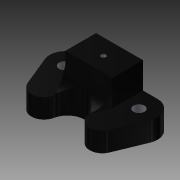
# Autodesk Inventor part: FrontStopper
Saved by Autodesk Inventor 2015 (Build 190159000, 159)
## iProperties
Created: 2017-01-04
Part Number: FrontStopper
Material: Generic
Document SubType Name: Modeling
Designer: Ernest
Density: 1 g/cm^3
Appearance: Default
Author: Ernest
Autodesk Inventor part; units mm, degrees
ref_plane "YZ Plane" through (0, 0, 0) normal (1, 0, 0) x (0, 1, 0)
ref_plane "XZ Plane" through (0, 0, 0) normal (0, 1, 0) x (-1, 0, 0)
ref_plane "XY Plane" through (0, 0, 0) normal (0, 0, 1) x (1, 0, 0)
sketch "Sketch1" plane through (0, 0, 0) normal (0, 0, 1) x (1, 0, 0)
  circle A0 centre (0, 0) radius 8
  circle A1 centre (25.5147, 5) radius 3
  circle A2 centre (-25.5147, 5) radius 3
  circle A3 centre (32.5, 30) radius 5
  circle A4 centre (-32.5, 30) radius 5
  arc A5 (45.4578, 24.6994) -> (32.5, 44) centre (32.5, 30) ccw
  arc A6 (-32.5, 44) -> (-45.4578, 24.6994) centre (-32.5, 30) ccw
  line L0 (-24.3676, 0) -> (22.7562, 0) construction
  line L1 (-38.3266, 30) -> (45.5284, 30) construction
  line L2 (-33.7528, 8) -> (48.0284, 8) construction
  circle A7 centre (-25.5147, 5) radius 6
  circle A8 centre (25.5147, 5) radius 6
  arc A9 (14.72, 2.8846) -> (-15, 0) centre (0, 0) ccw
  arc A10 (-35.6958, 0.8353) -> (-14.72, 2.8846) centre (-25.5147, 5) ccw
  arc A11 (14.72, 2.8846) -> (35.6958, 0.8353) centre (25.5147, 5) ccw
  line L3 (-45.4578, 24.6994) -> (-35.6958, 0.8353)
  line L4 (35.6958, 0.8353) -> (45.4578, 24.6994)
  line L5 (-32.5, 44) -> (32.5, 44)
  dimension "d0" = 65
  dimension "d1" = 32.5
  dimension "d2" = 10
  dimension "d3" = 10
  dimension "d4" = 6
  dimension "d5" = 6
  dimension "d6" = 28
  dimension "d7" = 28
  dimension "d14" = 16
  dimension "d16" = 15
  dimension "d18" = 12
  dimension "d19" = 12
  dimension "d20" = 30
  dimension "d33" = 30
  dimension "d34" = 15
  constraints: 12 centre point, 12 end point, 11 point on circle, 10 tangent, 8 coincident, 4 horizontal, 4 point on line, 2 parallel
  measures "d0" distance of A3.centre A4.centre
  measures "d1" horizontal distance of point (0, 0) A4.centre
  measures "d2" diameter of A4
  measures "d3" diameter of A3
  measures "d4" diameter of A2
  measures "d5" diameter of A1
  measures "d6" diameter of A5
  measures "d7" diameter of A6
  measures "d14" diameter of A0
  measures "d18" diameter of A7
  measures "d19" diameter of A8
  measures "d20" diameter of A9
  measures "d33" distance from line of point (0, 0) L1
extrude "Extrusion1" add sketch "Sketch1" along normal blind 12 contours L4 A11 A9 A10 L3 A6 L5 A5 | A7 | A8
sketch "Sketch2" plane through (0, 0, 12) normal (0, 0, 1) x (1, 0, 0)
  circle A0 centre (25.5147, 5) radius 3 projected
  circle A1 centre (-25.5147, 5) radius 3 projected
  circle A2 centre (-32.5, 30) radius 5 projected
  circle A3 centre (32.5, 30) radius 5 projected
  line L0 (-45.4578, 24.6994) -> (-35.6958, 0.8353) projected
  arc A4 (-35.6958, 0.8353) -> (-14.72, 2.8846) centre (-25.5147, 5) ccw projected
  arc A5 (14.72, 2.8846) -> (-14.72, 2.8846) centre (0, 0) ccw projected
  arc A6 (14.72, 2.8846) -> (35.6958, 0.8353) centre (25.5147, 5) ccw projected
  line L1 (35.6958, 0.8353) -> (45.4578, 24.6994) projected
  arc A7 (45.4578, 24.6994) -> (32.5, 44) centre (32.5, 30) ccw projected
  line L2 (32.5, 44) -> (-32.5, 44) projected
  arc A8 (-32.5, 44) -> (-45.4578, 24.6994) centre (-32.5, 30) ccw projected
  circle A9 centre (-32.5, 30) radius 5 projected
  circle A10 centre (-32.5, 30) radius 7.5
  circle A11 centre (32.5, 30) radius 5
  constraints: 2 centre point, 2 coincident, 1 concentric
extrude "Extrusion2" add sketch "Sketch2" along normal blind 5 contours A0 | A1 | A8 L2 A7 L1 A6 A5 A4 L0 | A10
sketch "Sketch3" plane through (0, 0, 17) normal (0, 0, 1) x (1, 0, 0)
  line L0 (-17.5, 40.5) -> (17.5, 40.5)
  line L1 (17.5, 40.5) -> (17.5, 18.5)
  line L2 (17.5, 18.5) -> (-17.5, 18.5)
  line L3 (-17.5, 18.5) -> (-17.5, 40.5)
  circle A0 centre (32.5, 30) radius 5 projected
  circle A1 centre (-32.5, 30) radius 5 projected
  line L4 (-45.4578, 24.6994) -> (-35.6958, 0.8353) projected
  arc A2 (-35.6958, 0.8353) -> (-14.72, 2.8846) centre (-25.5147, 5) ccw projected
  arc A3 (14.72, 2.8846) -> (-14.72, 2.8846) centre (0, 0) ccw projected
  arc A4 (14.72, 2.8846) -> (35.6958, 0.8353) centre (25.5147, 5) ccw projected
  line L5 (35.6958, 0.8353) -> (45.4578, 24.6994) projected
  arc A5 (45.4578, 24.6994) -> (32.5, 44) centre (32.5, 30) ccw projected
  line L6 (32.5, 44) -> (-32.5, 44) projected
  arc A6 (-32.5, 44) -> (-45.4578, 24.6994) centre (-32.5, 30) ccw projected
  dimension "d25" = 22
  dimension "d26" = 35
  dimension "d27" = 17.5
  dimension "d29" = 3.5
  dimension "d32" = 29
  constraints: 8 end point, 2 parallel, 1 horizontal, 1 perpendicular
  measures "d25" distance between parallel lines of L2 L0
  measures "d26" distance between parallel lines of L1 L3
  measures "d27" distance from line of point (0, 0) L3
  measures "d29" distance between parallel lines of L6 L0
  measures "d32" distance edge to line of A3 L6
extrude "Extrusion3" cut sketch "Sketch3" against normal blind 17 contours L0 L1 L2 L3
sketch "Sketch4" plane through (0, 0, 17) normal (0, 0, 1) x (1, 0, 0)
  line L0 (-17.5, 18.5) -> (-17.5, 40.5) projected
  line L1 (-17.5, 40.5) -> (17.5, 40.5) projected
  line L2 (17.5, 40.5) -> (17.5, 18.5) projected
  line L3 (17.5, 18.5) -> (-17.5, 18.5) projected
  circle A0 centre (32.5, 30) radius 5 projected
  circle A1 centre (-32.5, 30) radius 5 projected
  line L4 (-45.4578, 24.6994) -> (-35.6958, 0.8353) projected
  arc A2 (-35.6958, 0.8353) -> (-14.72, 2.8846) centre (-25.5147, 5) ccw projected
  arc A3 (14.72, 2.8846) -> (-14.72, 2.8846) centre (0, 0) ccw projected
  arc A4 (14.72, 2.8846) -> (35.6958, 0.8353) centre (25.5147, 5) ccw projected
  line L5 (35.6958, 0.8353) -> (45.4578, 24.6994) projected
  arc A5 (45.4578, 24.6994) -> (32.5, 44) centre (32.5, 30) ccw projected
  line L6 (32.5, 44) -> (-32.5, 44) projected
  arc A6 (-32.5, 44) -> (-45.4578, 24.6994) centre (-32.5, 30) ccw projected
  line L7 (32.5, 44) -> (-32.5, 44) projected
  line L8 (-20.5, 44) -> (20.5, 44)
  line L9 (20.5, 44) -> (20.5, 18.6633)
  line L10 (20.5, 18.6633) -> (-20.5, 18.6633)
  line L11 (-20.5, 18.6633) -> (-20.5, 44)
  arc A7 (14.72, 2.8846) -> (-14.72, 2.8846) centre (0, 0) ccw
  line L12 (-20.5, 18.6633) -> (-14.72, 2.8846)
  line L13 (20.5, 18.6633) -> (14.72, 2.8846)
  line L14 (-13, 39.5) -> (13, 39.5)
  line L15 (13, 39.5) -> (13, 23.5)
  line L16 (13, 23.5) -> (-13, 23.5)
  line L17 (-13, 23.5) -> (-13, 39.5)
  dimension "d35" = 3
  dimension "d36" = 3
  dimension "d37" = 26
  dimension "d38" = 16
  dimension "d39" = 1
  dimension "d40" = 4.5
  constraints: 20 end point, 4 parallel, 2 horizontal, 2 perpendicular, 2 point on circle, 1 centre point, 1 coincident, 1 point on line
  measures "d35" distance between parallel lines of L9 L2
  measures "d36" distance between parallel lines of L0 L11
  measures "d37" distance of L14.start L14.end
  measures "d38" distance of L14.end L15.end
  measures "d39" distance between parallel lines of L1 L14
  measures "d40" distance between parallel lines of L17 L0
extrude "Extrusion4" add sketch "Sketch4" along normal blind 13 contours L3 L2 L10 L13 A3 L12 L0 | L0 L10 L2 L3 | L10 L11 L6 L9 L2 L1 L0 | L0 L1 L2 L10
sketch "Sketch5" plane through (20.5, 18.6633, 17) normal (1, 0, 0) x (0, 0, -1)
  line L0 (0, 25.3367) -> (0, 0) projected
  line L1 (0, 25.3367) -> (-13, 25.3367) projected
  line L2 (-13, 0) -> (-13, 25.3367) projected
  line L3 (0, 0) -> (-13, 0) projected
  line L4 (0, 0) -> (0, -15.7787) projected
  line L5 (0, 0) -> (-13, 0) projected
  line L6 (-13, -15.7787) -> (-13, 0) projected
  line L7 (0, -15.7787) -> (-13, -15.7787) projected
  arc A0 (0, -15.7787) -> (-13, 0) centre (-19.7674, -18.8203) ccw
  line L8 (-13, 0) -> (-13, -15.7787)
  line L9 (-13, -15.7787) -> (0, -15.7787)
  point P0 (17, -18.6633)
  dimension "d43" = 20
  constraints: 4 end point, 2 point on circle, 1 centre point, 1 collinear, 1 perpendicular
  measures "d43" radius of A0
extrude "Extrusion5" cut sketch "Sketch5" against normal blind 67 contours A0 L7 L6
sketch "Sketch6" plane through (0, 0, 30) normal (0, 0, 1) x (1, 0, 0)
  line L0 (-20.5, 18.6633) -> (20.5, 18.6633) projected
  line L1 (20.5, 18.6633) -> (20.5, 44) projected
  line L2 (20.5, 44) -> (-20.5, 44) projected
  line L3 (-20.5, 44) -> (-20.5, 18.6633) projected
  line L4 (13, 39.5) -> (13, 23.5) projected
  line L5 (13, 23.5) -> (-13, 23.5) projected
  line L6 (-13, 23.5) -> (-13, 39.5) projected
  line L7 (-13, 39.5) -> (13, 39.5) projected
  line L8 (-20.5, 44) -> (20.5, 44)
  line L9 (20.5, 44) -> (20.5, 18.6633)
  line L10 (20.5, 18.6633) -> (-20.5, 18.6633)
  line L11 (-20.5, 18.6633) -> (-20.5, 44)
  circle A0 centre (0, 31.5) radius 2
  point P0 (0, 0)
  dimension "d46" = 16
  dimension "d47" = 26
  dimension "d50" = 8
  dimension "d51" = 13
  dimension "d52" = 4
  constraints: 8 end point, 2 parallel, 1 centre point, 1 horizontal, 1 perpendicular
  measures "d46" distance of L5.end L6.end
  measures "d47" distance of L6.end L4.start
  measures "d50" distance from line of L5 A0.centre
  measures "d51" distance from line of L6 A0.centre
  measures "d52" diameter of A0
extrude "Extrusion6" add sketch "Sketch6" along normal blind 10 contours L3 L2 L1 L0 | L4 L5 L6 L7
sketch "Sketch7" plane through (0, 0, 0) normal (0, 0, -1) x (-1, 0, 0)
  line L0 (17.5, 40.5) -> (17.5, 18.5) projected
  line L1 (17.5, 18.5) -> (-17.5, 18.5) projected
  line L2 (-17.5, 18.5) -> (-17.5, 40.5) projected
  line L3 (-17.5, 40.5) -> (17.5, 40.5) projected
  circle A0 centre (-25.5147, 5) radius 3 projected
  circle A1 centre (25.5147, 5) radius 3 projected
  circle A2 centre (32.5, 30) radius 5 projected
  circle A3 centre (-32.5, 30) radius 5 projected
  line L4 (35.6958, 0.8353) -> (45.4578, 24.6994) projected
  arc A4 (45.4578, 24.6994) -> (32.5, 44) centre (32.5, 30) ccw projected
  line L5 (32.5, 44) -> (-32.5, 44) projected
  arc A5 (-32.5, 44) -> (-45.4578, 24.6994) centre (-32.5, 30) ccw projected
  line L6 (-45.4578, 24.6994) -> (-35.6958, 0.8353) projected
  arc A6 (-35.6958, 0.8353) -> (-14.72, 2.8846) centre (-25.5147, 5) ccw projected
  arc A7 (14.72, 2.8846) -> (-14.72, 2.8846) centre (0, 0) ccw projected
  arc A8 (14.72, 2.8846) -> (35.6958, 0.8353) centre (25.5147, 5) ccw projected
  line L7 (-33.1666, 45.5) -> (33.5331, 45.5)
  arc A9 (-32.5, 44) -> (-45.4578, 24.6994) centre (-32.5, 30) ccw projected
  arc A10 (-33.1666, 45.5) -> (-45.7516, 25.4839) centre (-33.1666, 31.5356) ccw
  arc A11 (45.4578, 24.6994) -> (32.5, 44) centre (32.5, 30) ccw projected
  arc A12 (45.8112, 25.6626) -> (33.5331, 45.5) centre (33.5331, 31.7816) ccw
  dimension "d55" = 5
  constraints: 8 point on circle, 4 tangent, 2 centre point, 2 end point, 1 horizontal
  measures "d55" distance between parallel lines of L3 L7
extrude "Extrusion7" add sketch "Sketch7" against normal blind 17 contours A4 L5 A5 A10 L7 A12
sketch "Sketch8" plane through (-20.5, 44, 17) normal (0, 1, 0) x (1, 0, 0)
  line L0 (41, 0) -> (0, 0) projected
  line L1 (0, 0) -> (0, -23) projected
  line L2 (41, -23) -> (0, -23) projected
  line L3 (41, 0) -> (41, -23) projected
  point P0 (20.5, 17)
extrude "Extrusion8" add sketch "Sketch8" along normal blind 1.5
sketch "Sketch9" plane through (0, 0, 0) normal (0, 0, -1) x (-1, 0, 0)
  line L0 (17.5, 40.5) -> (17.5, 18.5) projected
  line L1 (17.5, 18.5) -> (-17.5, 18.5) projected
  line L2 (-17.5, 18.5) -> (-17.5, 40.5) projected
  line L3 (-17.5, 40.5) -> (17.5, 40.5) projected
  circle A0 centre (-25.5147, 5) radius 3 projected
  circle A1 centre (25.5147, 5) radius 3 projected
  circle A2 centre (32.5, 30) radius 5 projected
  circle A3 centre (-32.5, 30) radius 5 projected
  line L4 (35.6958, 0.8353) -> (45.4578, 24.6994) projected
  arc A4 (45.4578, 24.6994) -> (45.8112, 25.6626) centre (32.5, 30) ccw projected
  arc A5 (45.8112, 25.6626) -> (33.5331, 45.5) centre (33.5331, 31.7816) ccw projected
  line L5 (33.5331, 45.5) -> (-33.1666, 45.5) projected
  arc A6 (-33.1666, 45.5) -> (-45.7516, 25.4839) centre (-33.1666, 31.5356) ccw projected
  arc A7 (-45.7516, 25.4839) -> (-45.4578, 24.6994) centre (-32.5, 30) ccw projected
  line L6 (-45.4578, 24.6994) -> (-35.6958, 0.8353) projected
  arc A8 (-35.6958, 0.8353) -> (-14.72, 2.8846) centre (-25.5147, 5) ccw projected
  arc A9 (14.72, 2.8846) -> (-14.72, 2.8846) centre (0, 0) ccw projected
  arc A10 (14.72, 2.8846) -> (35.6958, 0.8353) centre (25.5147, 5) ccw projected
  circle A11 centre (-25.5147, 5) radius 3.2
  circle A12 centre (25.5147, 5) radius 3.2
  circle A13 centre (32.5, 30) radius 4.75
  circle A14 centre (-32.5, 30) radius 4.75
  dimension "d60" = 6.4
  dimension "d61" = 6.4
  dimension "d62" = 9.5
  dimension "d63" = 9.5
  constraints: 4 centre point, 4 coincident
  measures "d60" diameter of A11
  measures "d61" diameter of A12
  measures "d62" diameter of A13
  measures "d63" diameter of A14
extrude "Extrusion9" add sketch "Sketch9" against normal up to surface (17 mm away) contours A2 | A3
extrude "Extrusion10" cut sketch "Sketch9" against normal up to surface (12 mm away) contours A11 | A12
equation "\"d1\" = 0.5 * d0"
equation "\"d27\" = 0.5 * d26"
equation "\"d29\" = 0.5 * d32 - 0.5 * d25"
equation "\"d50\" = 0.5 * d46"
equation "\"d51\" = 0.5 * d47"
body "Solid1"
